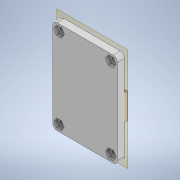
# Autodesk Inventor part: bottom
Saved by Autodesk Inventor 2021.2 (Build 252289000, 289)
## iProperties
Created: 2021-11-19
Part Number: bottom
Material: Типовые
Document SubType Name: Modeling
Designer: kanad
Density: 1 g/cm^3
Appearance: По умолчанию
Author: kanad
Autodesk Inventor part; units mm, degrees
ref_plane "YZ Plane" through (0, 0, 0) normal (1, 0, 0) x (0, 1, 0)
ref_plane "XZ Plane" through (0, 0, 0) normal (0, 1, 0) x (-1, 0, 0)
ref_plane "XY Plane" through (0, 0, 0) normal (0, 0, 1) x (1, 0, 0)
ref_plane "РабПлоскость1" through (0, 0, 0) normal (0, 0, 1) x (1, 0, 0)
sketch "Эскиз1" plane through (0, 0, 0) normal (0, 0, 1) x (1, 0, 0)
  line L0 (22.5, 29.5) -> (22.5, 9) projected
  arc A0 (22.5, 29.5) -> (19.5, 32.5) centre (19.5, 29.5) ccw projected
  line L1 (-19.5, 32.5) -> (19.5, 32.5) projected
  arc A1 (-19.5, 32.5) -> (-22.5, 29.5) centre (-19.5, 29.5) ccw projected
  line L2 (-22.5, -29.5) -> (-22.5, 29.5) projected
  arc A2 (-22.5, -29.5) -> (-19.5, -32.5) centre (-19.5, -29.5) ccw projected
  line L3 (19.5, -32.5) -> (-19.5, -32.5) projected
  arc A3 (19.5, -32.5) -> (22.5, -29.5) centre (19.5, -29.5) ccw projected
  line L4 (22.5, -9) -> (22.5, -29.5) projected
  line L5 (20, -9) -> (22.5, -9) projected
  line L6 (20, -25) -> (20, -9) projected
  line L7 (18, -25) -> (20, -25) projected
  arc A4 (18, -25) -> (15, -28) centre (18, -28) ccw projected
  line L8 (15, -30) -> (15, -28) projected
  line L9 (-15, -30) -> (15, -30) projected
  line L10 (-15, -28) -> (-15, -30) projected
  arc A5 (-15, -28) -> (-18, -25) centre (-18, -28) ccw projected
  line L11 (-20, -25) -> (-18, -25) projected
  line L12 (-20, 25) -> (-20, -25) projected
  line L13 (-18, 25) -> (-20, 25) projected
  arc A6 (-18, 25) -> (-15, 28) centre (-18, 28) ccw projected
  line L14 (-15, 30) -> (-15, 28) projected
  line L15 (15, 30) -> (-15, 30) projected
  line L16 (15, 28) -> (15, 30) projected
  arc A7 (15, 28) -> (18, 25) centre (18, 28) ccw projected
  line L17 (20, 25) -> (18, 25) projected
  line L18 (20, 9) -> (20, 25) projected
  line L19 (22.5, 9) -> (20, 9) projected
  circle A8 centre (-18, -28) radius 1.5 projected
  circle A9 centre (-18, 28) radius 1.5 projected
  circle A10 centre (18, 28) radius 1.5 projected
  circle A11 centre (18, -28) radius 1.5 projected
  line L20 (22.5, 9) -> (22.5, -9)
  line L21 (20, 9) -> (20, -9.6142)
  circle A12 centre (18, 28) radius 4.2426
  circle A13 centre (18, -28) radius 4.2426
  circle A14 centre (-18, -28) radius 4.2426
  circle A15 centre (-18, 28) radius 4.2426
  point P0 (0, 0)
  point P1 (-14.2583, -30)
  point P2 (-20, -24.2583)
  point P3 (-20, 24.2583)
  point P4 (-14.2583, 30)
  point P5 (20, -24.2583)
  point P6 (14.2583, -30)
  point P7 (14.2583, 30)
  point P8 (20, 24.2583)
  constraints: 4 centre point, 4 coincident, 4 end point, 1 point on line, 1 vertical
extrude "Выдавливание1" add sketch "Эскиз1" along normal blind 4 contours L0 L19 L18 A12 L15 A15 L12 A14 L9 A13 L6 L5 L4 A3 L3 A2 L2 A1 L1 A0 | L20 L5 L21 L19 | A12 L15 L16 A7 L17 L18 | L18 L17 A7 L16 L15 A12 | A15 L12 L13 A6 L14 L15 | L15 L14 A6 L13 L12 A15 | A13 L9 L8 A4 L7 L6 | L6 L7 A4 L8 L9 A13 | A14 L9 L10 A5 L11 L12 | L12 L11 A5 L10 L9 A14
sketch "Эскиз2" plane through (0, 0, 4) normal (0, 0, 1) x (1, 0, 0)
  circle A0 centre (18, 28) radius 1.5 projected
  circle A1 centre (18, -28) radius 1.5 projected
  circle A2 centre (-18, 28) radius 1.5 projected
  line L0 (16.1813, 24.85) -> (14.3627, 28)
  line L1 (14.3627, 28) -> (16.1813, 31.15)
  line L2 (16.1813, 31.15) -> (19.8187, 31.15)
  line L3 (19.8187, 31.15) -> (21.6373, 28)
  line L4 (21.6373, 28) -> (19.8187, 24.85)
  line L5 (19.8187, 24.85) -> (16.1813, 24.85)
  circle A3 centre (18, -28) radius 1.5 projected
  line L6 (21.6373, -28) -> (19.8187, -31.15)
  line L7 (19.8187, -31.15) -> (16.1813, -31.15)
  line L8 (16.1813, -31.15) -> (14.3627, -28)
  line L9 (14.3627, -28) -> (16.1813, -24.85)
  line L10 (16.1813, -24.85) -> (19.8187, -24.85)
  line L11 (19.8187, -24.85) -> (21.6373, -28)
  line L12 (-14.3627, 28.0054) -> (-16.1766, 24.8527)
  line L13 (-16.1766, 24.8527) -> (-19.8139, 24.8473)
  line L14 (-19.8139, 24.8473) -> (-21.6373, 27.9946)
  line L15 (-21.6373, 27.9946) -> (-19.8234, 31.1473)
  line L16 (-19.8234, 31.1473) -> (-16.1861, 31.1527)
  line L17 (-16.1861, 31.1527) -> (-14.3627, 28.0054)
  line L18 (-16.2701, -24.9933) -> (-14.5312, -27.9948)
  line L19 (-14.5312, -27.9948) -> (-16.2611, -31.0015)
  line L20 (-16.2611, -31.0015) -> (-19.7299, -31.0067)
  line L21 (-19.7299, -31.0067) -> (-21.4688, -28.0052)
  line L22 (-21.4688, -28.0052) -> (-19.7389, -24.9985)
  line L23 (-19.7389, -24.9985) -> (-16.2701, -24.9933)
  line L24 (19.5, 32.5) -> (-19.5, 32.5) projected
  point P0 (0, 0)
  point P1 (-18, -28)
  point P2 (-18, -28)
  dimension "d2" = 6.3
  constraints: 48 end point, 4 coincident, 2 equal length, 2 parallel, 52 other
  measures "d2" distance between parallel lines of L5 L2
sketch "Эскиз3" plane through (0, 0, 4) normal (0, 0, 1) x (1, 0, 0)
  line L0 (19.5, 32.5) -> (-19.5, 32.5) projected
  arc A0 (22.5, 29.5) -> (19.5, 32.5) centre (19.5, 29.5) ccw projected
  line L1 (22.5, -29.5) -> (22.5, 29.5) projected
  arc A1 (19.5, -32.5) -> (22.5, -29.5) centre (19.5, -29.5) ccw projected
  line L2 (-19.5, -32.5) -> (19.5, -32.5) projected
  arc A2 (-22.5, -29.5) -> (-19.5, -32.5) centre (-19.5, -29.5) ccw projected
  line L3 (-22.5, 29.5) -> (-22.5, -29.5) projected
  arc A3 (-19.5, 32.5) -> (-22.5, 29.5) centre (-19.5, 29.5) ccw projected
  point P0 (0, 0)
extrude "Выдавливание2" add sketch "Эскиз3" along normal blind 1
extrude "Выдавливание3" cut sketch "Эскиз2" along normal blind 1 and the other way blind 1.25 contours A0 | A1 | A2 | L0 L1 L2 L3 L4 L5 | L6 L7 L8 L9 L10 L11 | L12 L13 L14 L15 L16 L17 | L18 L19 L20 L21 L22 L23
sketch "Эскиз4" plane through (0, 0, 0) normal (0, 0, -1) x (-1, 0, 0)
  line L0 (-20.25, -30.25) -> (20.25, -30.25)
  line L1 (20.25, -30.25) -> (20.25, 30.25)
  line L2 (20.25, 30.25) -> (-20.25, 30.25)
  line L3 (-20.25, 30.25) -> (-20.25, -30.25)
  line L4 (-20.25, -30.25) -> (20.25, 30.25) construction
  line L5 (20.25, -30.25) -> (-20.25, 30.25) construction
  point P0 (0, 0)
  dimension "d9" = 40.5
  dimension "d10" = 60.5
  constraints: 12 end point, 2 midpoint, 2 parallel, 1 horizontal, 1 perpendicular
  measures "d9" distance of L2.end L1.end
  measures "d10" distance of L1.end L0.end
extrude "Выдавливание4" cut sketch "Эскиз4" against normal blind 1.6
sketch "Эскиз5" plane through (0, 0, 0) normal (0, 0, -1) x (-1, 0, 0)
  line L0 (-20, 9) -> (-20, -9) projected
  line L1 (-22.5, 29.5) -> (-22.5, -29.5) projected
  line L2 (-22.5, -29.5) -> (-22.5, 29.5) projected
  line L3 (-20, 9) -> (-22.5, 9)
  line L4 (-22.5, 9) -> (-22.5, -9)
  line L5 (-22.5, -9) -> (-20, -9)
  line L6 (-20, -9) -> (-20, 9)
  point P0 (0, 0)
  constraints: 8 end point, 2 parallel, 1 horizontal, 1 perpendicular, 1 point on line
extrude "Выдавливание5" add sketch "Эскиз5" along normal blind 1.85
